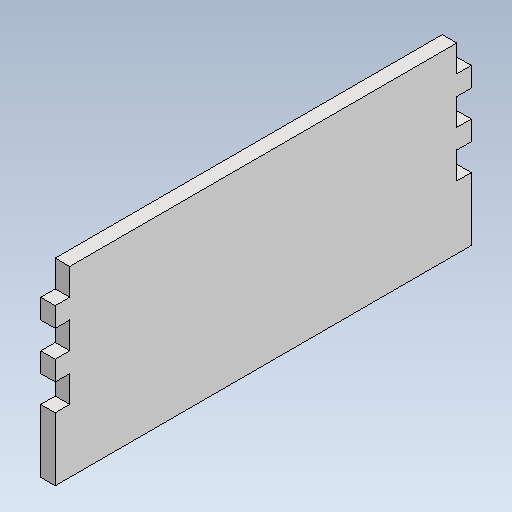
# Autodesk Inventor part: gate
Saved by Autodesk Inventor 2025 (Build 290162000, 162)
## iProperties
Created: 2025-08-22
Part Number: gate
Material: Generic
Document SubType Name: Modeling
Designer: HP
Density: 1 g/cm^3
Appearance: Default
Author: HP
Autodesk Inventor part; units mm, degrees
ref_plane "YZ Plane" through (0, 0, 0) normal (1, 0, 0) x (0, 1, 0)
ref_plane "XZ Plane" through (0, 0, 0) normal (0, 1, 0) x (-1, 0, 0)
ref_plane "XY Plane" through (0, 0, 0) normal (0, 0, 1) x (1, 0, 0)
sketch "Sketch1" plane through (0, 0, 0) normal (1, 0, 0) x (0, 1, 0)
  line L0 (-31.5, 71.75) -> (31.5, 71.75)
  line L1 (31.5, 71.75) -> (31.5, -71.75)
  line L2 (31.5, -71.75) -> (-31.5, -71.75)
  line L3 (-31.5, -71.75) -> (-31.5, 71.75)
  line L4 (-31.5, 71.75) -> (31.5, -71.75) construction
  line L5 (31.5, 71.75) -> (-31.5, -71.75) construction
  line L6 (12.4, 71.75) -> (24.4, 71.75)
  line L7 (6.3, 71.75) -> (15.5, 71.75)
  line L8 (15.5, 71.75) -> (15.5, 66.75)
  line L9 (15.5, 66.75) -> (6.3, 66.75)
  line L10 (6.3, 66.75) -> (6.3, 71.75)
  line L11 (6.3, 71.75) -> (15.5, 66.75) construction
  line L12 (15.5, 71.75) -> (6.3, 66.75) construction
  line L13 (22.3, 66.75) -> (31.5, 66.75)
  line L14 (31.5, 66.75) -> (31.5, 71.75)
  line L15 (31.5, 71.75) -> (22.3, 71.75)
  line L16 (22.3, 71.75) -> (22.3, 66.75)
  line L17 (22.3, 66.75) -> (31.5, 71.75) construction
  line L18 (31.5, 66.75) -> (22.3, 71.75) construction
  line L19 (-9.7, 71.75) -> (-0.5, 71.75)
  line L20 (-0.5, 71.75) -> (-0.5, 66.75)
  line L21 (-0.5, 66.75) -> (-9.7, 66.75)
  line L22 (-9.7, 66.75) -> (-9.7, 71.75)
  line L23 (-9.7, 71.75) -> (-0.5, 66.75) construction
  line L24 (-0.5, 71.75) -> (-9.7, 66.75) construction
  point P0 (0, 0)
  point P1 (10.9, 69.25)
  point P2 (26.9, 69.25)
  point P3 (31.5, 69.25)
  point P4 (22.3, 71.75)
  point P5 (-5.1, 69.25)
  point P6 (-0.5, 71.75)
  dimension "d0" = 143.5
  dimension "d1" = 63
  dimension "d19" = 5
  dimension "d20" = 9.2
  dimension "d21" = 9.2
  dimension "d22" = 5
  dimension "d23" = 16
  dimension "d26" = 6.8
  dimension "d27" = 16
  dimension "d28" = 9.2
  constraints: 50 end point, 9 midpoint, 8 parallel, 5 horizontal, 4 collinear, 4 perpendicular
  measures "d0" distance between parallel lines of L2 L0
  measures "d1" distance between parallel lines of L3 L1
  measures "d19" distance between parallel lines of L13 L15
  measures "d20" distance from line of L16 point (31.5, 69.25)
  measures "d21" distance between parallel lines of L10 L8
  measures "d22" distance between parallel lines of L7 L9
  measures "d23" distance of point (10.9, 69.25) point (26.9, 69.25)
  measures "d26" distance between parallel lines of L8 L16
  measures "d27" distance of point (10.9, 69.25) point (-5.1, 69.25)
  measures "d28" distance between parallel lines of L22 L20
extrude "Extrusion1" add sketch "Sketch1" along normal blind 5
extrude "Extrusion3" cut sketch "Sketch1" along normal through all contours L0 L20 L21 L22 | L0 L8 L9 L10 | L13 L16 L0 L1
mirror "Mirror1" about plane through (0, 0, 0) normal (0, 0, 1) of "Extrusion3"
equation "\"d21\" = d20"
equation "\"d22\" = d19"
equation "\"d27\" = d23"
equation "\"d28\" = d21"
body "Solid1"
